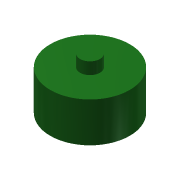
# Autodesk Inventor part: 滾輪
Saved by Autodesk Inventor 2015 SP2 (Build 190223200, 223)
## iProperties
Created: 2020-03-26
Part Number: 滾輪
Material: 一般
Document SubType Name: Modeling
Designer: Kuan-Lun Hsu
Density: 1 g/cm^3
Appearance: 平滑 - 深森林綠
Mass: 3.2594 g
Surface Area: 13.5088 cm^2
Volume: 3.2594 cm^3
Author: Kuan-Lun Hsu
Autodesk Inventor part; units mm, degrees
ref_plane "YZ Plane" through (0, 0, 0) normal (1, 0, 0) x (0, 1, 0)
ref_plane "XZ Plane" through (0, 0, 0) normal (0, 1, 0) x (-1, 0, 0)
ref_plane "XY Plane" through (0, 0, 0) normal (0, 0, 1) x (1, 0, 0)
sketch "草圖1" plane through (0, 0, 0) normal (0, 0, 1) x (1, 0, 0)
  circle A0 centre (0, 0) radius 10
  dimension "d0" = 20
  constraints: 1 centre point, 1 coincident
  measures "d0" diameter of A0
extrude "擠出1" add sketch "草圖1" along normal mid plane 10
sketch "草圖2" plane through (0, 0, 5) normal (0, 0, 1) x (1, 0, 0)
  circle A0 centre (0, 0) radius 2.5
  dimension "d3" = 5
  constraints: 1 centre point, 1 coincident
  measures "d3" diameter of A0
extrude "擠出2" add sketch "草圖2" along normal blind 3
mirror "鏡射1" about plane through (0, 0, 0) normal (0, 0, 1) of "擠出2"
